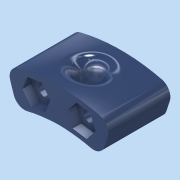
# Autodesk Inventor part: carriage
Saved by Autodesk Inventor 2017 (Build 210142000, 142)
## iProperties
Created: 2016-12-14
Part Number: carriage
Material: ABS Plastic
Document SubType Name: Modeling
Designer: techn
Density: 1.06 g/cm^3
Appearance: Flaked Satin - Blue
Author: techn
Autodesk Inventor part; units mm, degrees
ref_plane "YZ Plane" through (0, 0, 0) normal (1, 0, 0) x (0, 1, 0)
ref_plane "XY Plane" through (0, 0, 0) normal (0, 0, 1) x (1, 0, 0)
sketch "Sketch1" plane through (0, 0, 0) normal (0, 0, 1) x (1, 0, 0)
  circle A0 centre (0, 0) radius 50.8
  line L0 (0, 0) -> (6.35, 42.3253)
  line L1 (6.35, 42.3253) -> (-6.35, 42.3253)
  line L2 (-6.35, 42.3253) -> (0, 0)
  line L3 (0, 0) -> (-15.6981, 48.3137)
  line L4 (0, 0) -> (50.8, 0) construction
  line L5 (0, 0) -> (15.6981, 48.3137)
  line L6 (0, 0) -> (50.8, 0) construction
  line L7 (3.8834, 39.228) -> (2.4344, 42.9128)
  line L8 (2.4344, 42.9128) -> (4.9009, 46.0101)
  line L9 (4.9009, 46.0101) -> (8.8166, 45.4226)
  line L10 (8.8166, 45.4226) -> (10.2656, 41.7379)
  line L11 (10.2656, 41.7379) -> (7.7991, 38.6405)
  line L12 (7.7991, 38.6405) -> (3.8834, 39.228)
  arc A1 (11.7735, 36.2353) -> (-11.7735, 36.2353) centre (0, 0) ccw
  arc A2 (14.7169, 45.2941) -> (-14.7169, 45.2941) centre (0, 0) ccw
  line L13 (-2.4344, 42.9128) -> (-3.8834, 39.228)
  line L14 (-3.8834, 39.228) -> (-7.7991, 38.6405)
  line L15 (-7.7991, 38.6405) -> (-10.2656, 41.7379)
  line L16 (-10.2656, 41.7379) -> (-8.8166, 45.4226)
  line L17 (-8.8166, 45.4226) -> (-4.9009, 46.0101)
  line L18 (-4.9009, 46.0101) -> (-2.4344, 42.9128)
  dimension "d0" = 101.6
  dimension "d1" = 42.799
  dimension "d2" = 12.7
  dimension "d3" = 42.799
  dimension "d6" = 50.8
  dimension "d7" = 108
  dimension "d8" = 50.8
  dimension "d9" = 72
  dimension "d10" = 6.858
  dimension "d11" = 38.1
  dimension "d12" = 47.625
  dimension "d32" = 6.858
  constraints: 38 end point, 6 coincident, 4 point on circle, 4 point on line, 3 centre point, 3 horizontal, 2 equal length, 2 perpendicular, 26 other
  measures "d0" diameter of A0
  measures "d1" distance of L0.start L0.end
  measures "d2" distance of L0.end L1.end
  measures "d3" distance of L1.end L0.start
  measures "d6" distance of L0.start L3.end
  measures "d7" angle of L4 L3
  measures "d8" distance of L0.start L5.end
  measures "d9" angle of L6 L5
  measures "d10" distance between parallel lines of L11 L8
  measures "d11" radius of A1
  measures "d12" radius of A2
  measures "d32" distance between parallel lines of L14 L17
extrude "Extrusion8" add sketch "Sketch1" along normal blind 2.3813 contours L5 A1 L0 L12 L11 L10 L9 L8 L7 L1 L13 L18 L17 L16 L15 L14 L2 L3 A2 | A1 L2 L14 L13 L1 L7 L12 L0
sketch "Sketch8" plane through (0, 0, 2.3813) normal (0, 0, 1) x (1, 0, 0)
  line L0 (-3.8834, 39.228) -> (-7.7991, 38.6405) projected
  line L1 (-7.7991, 38.6405) -> (-10.2656, 41.7379) projected
  line L2 (-10.2656, 41.7379) -> (-8.8166, 45.4226) projected
  line L3 (-8.8166, 45.4226) -> (-4.9009, 46.0101) projected
  line L4 (-4.9009, 46.0101) -> (-2.4344, 42.9128) projected
  line L5 (-2.4344, 42.9128) -> (-3.8834, 39.228) projected
  line L6 (2.4344, 42.9128) -> (4.9009, 46.0101) projected
  line L7 (4.9009, 46.0101) -> (8.8166, 45.4226) projected
  line L8 (8.8166, 45.4226) -> (10.2656, 41.7379) projected
  line L9 (10.2656, 41.7379) -> (7.7991, 38.6405) projected
  line L10 (7.7991, 38.6405) -> (3.8834, 39.228) projected
  line L11 (3.8834, 39.228) -> (2.4344, 42.9128) projected
  line L12 (11.7735, 36.2353) -> (14.7169, 45.2941) projected
  arc A0 (14.7169, 45.2941) -> (-14.7169, 45.2941) centre (0, 0) ccw projected
  line L13 (-14.7169, 45.2941) -> (-11.7735, 36.2353) projected
  arc A1 (11.7735, 36.2353) -> (-11.7735, 36.2353) centre (0, 0) ccw projected
extrude "Extrusion9" add sketch "Sketch8" along normal blind 12.7 contours L0 L1 L2 L3 L4 L5 | L6 L7 L8 L9 L10 L11 | A1 L13 A0 L12
sketch "Sketch9" plane through (0, 0, 15.0813) normal (0, 0, 1) x (1, 0, 0)
  line L0 (-7.7991, 38.6405) -> (-3.8834, 39.228) projected
  line L1 (-3.8834, 39.228) -> (-2.4344, 42.9128) projected
  line L2 (-2.4344, 42.9128) -> (-4.9009, 46.0101) projected
  line L3 (-4.9009, 46.0101) -> (-8.8166, 45.4226) projected
  line L4 (-8.8166, 45.4226) -> (-10.2656, 41.7379) projected
  line L5 (-10.2656, 41.7379) -> (-7.7991, 38.6405) projected
  line L6 (4.9009, 46.0101) -> (2.4344, 42.9128) projected
  line L7 (2.4344, 42.9128) -> (3.8834, 39.228) projected
  line L8 (3.8834, 39.228) -> (7.7991, 38.6405) projected
  line L9 (7.7991, 38.6405) -> (10.2656, 41.7379) projected
  line L10 (10.2656, 41.7379) -> (8.8166, 45.4226) projected
  line L11 (8.8166, 45.4226) -> (4.9009, 46.0101) projected
  line L12 (11.7735, 36.2353) -> (14.7169, 45.2941) projected
  arc A0 (11.7735, 36.2353) -> (-11.7735, 36.2353) centre (0, 0) ccw projected
  line L13 (-14.7169, 45.2941) -> (-11.7735, 36.2353) projected
  arc A1 (14.7169, 45.2941) -> (-14.7169, 45.2941) centre (0, 0) ccw projected
extrude "Extrusion10" add sketch "Sketch9" along normal blind 2.3813
sketch "Sketch10" plane through (0, 0, 17.4625) normal (0, 0, 1) x (1, 0, 0)
  line L0 (-10.2656, 41.7379) -> (-7.7991, 38.6405) projected
  line L1 (-7.7991, 38.6405) -> (-3.8834, 39.228) projected
  line L2 (-3.8834, 39.228) -> (-2.4344, 42.9128) projected
  line L3 (-2.4344, 42.9128) -> (-4.9009, 46.0101) projected
  line L4 (-4.9009, 46.0101) -> (-8.8166, 45.4226) projected
  line L5 (-8.8166, 45.4226) -> (-10.2656, 41.7379) projected
  line L6 (8.8166, 45.4226) -> (4.9009, 46.0101) projected
  line L7 (4.9009, 46.0101) -> (2.4344, 42.9128) projected
  line L8 (2.4344, 42.9128) -> (3.8834, 39.228) projected
  line L9 (3.8834, 39.228) -> (7.7991, 38.6405) projected
  line L10 (7.7991, 38.6405) -> (10.2656, 41.7379) projected
  line L11 (10.2656, 41.7379) -> (8.8166, 45.4226) projected
  circle A0 centre (-6.35, 42.3253) radius 1.778
  circle A1 centre (6.35, 42.3253) radius 1.778
  point P0 (0, 0)
  dimension "d39" = 3.556
  dimension "d40" = 3.556
  constraints: 2 centre point
  measures "d39" diameter of A0
  measures "d40" diameter of A1
extrude "Extrusion11" cut sketch "Sketch10" against normal through all contours A0 | A1
ref_plane "Work Plane3" through (0, 47.625, 0) normal (0, 1, 0) x (-1, 0, 0)
sketch "Sketch11" plane through (0, 47.625, 0) normal (0, 1, 0) x (-1, 0, 0)
  line L0 (-14.7169, 0) -> (14.7169, 0) projected
  line L1 (14.7169, 0) -> (14.7169, 17.4625) projected
  line L2 (-14.7169, 17.4625) -> (14.7169, 17.4625) projected
  line L3 (-14.7169, 0) -> (-14.7169, 17.4625) projected
  circle A0 centre (0, 8.7313) radius 3.175
  point P0 (0, 0)
  dimension "d43" = 6.35
  dimension "d48" = 8.7312
  dimension "d49" = 17.4625
  constraints: 1 centre point
  measures "d43" diameter of A0
  measures "d48" distance from line of L0 A0.centre
  measures "d49" distance between parallel lines of L2 L0
extrude "Extrusion12" cut sketch "Sketch11" against normal through all contours A0
fillet "Fillet2" radius 6.35 1 edges at (3.1628, 37.9685, 8.4534)
fillet "Fillet3" radius 3.175 3 edges at (3.175, 47.519, 8.7323) (-2.2621, 47.5712, 10.9592) (-2.418, 47.5636, 6.6736)
fillet "Fillet4" radius 3.175 4 edges at (-11.7735, 36.2353, 8.7313) (-14.7169, 45.2941, 8.7313) (11.7735, 36.2353, 8.7313) (14.7169, 45.2941, 8.7313)
equation "\"d3\" = d1"
equation "\"d48\" = 0.5 * d49"
body "Solid2"
